Autodesk Fusion 360 part; units mm, degrees
note: some values were not read from the file. Set by a fixed rule: which sketch regions a step uses.
(part 3 of 3)
  arc A1078 (120.8139, 18.409) -> (120.8089, 18.409) centre (120.8114, 18.409) ccw
  arc A1079 (117.7319, 17.663) -> (117.7269, 17.663) centre (117.7294, 17.663) ccw
  arc A1080 (118.5519, 18.189) -> (118.5469, 18.189) centre (118.5494, 18.189) ccw
  arc A1081 (117.9059, 17.837) -> (117.9009, 17.837) centre (117.9034, 17.837) ccw
  arc A1082 (118.7879, 18.242) -> (118.7929, 18.242) centre (118.7904, 18.242) ccw
  arc A1083 (120.8089, 18.409) -> (120.8139, 18.409) centre (120.8114, 18.409) ccw
  arc A1084 (118.5469, 18.189) -> (118.5519, 18.189) centre (118.5494, 18.189) ccw
  line L282 (118.7904, 18.242) -> (119.0274, 18.259)
  line L283 (119.0274, 18.259) -> (119.0364, 18.255)
  arc A1085 (117.4659, 17.248) -> (117.4609, 17.248) centre (117.4634, 17.248) ccw
  line L284 (117.9034, 17.837) -> (118.1014, 17.985)
  arc A1086 (118.3159, 18.103) -> (118.3209, 18.103) centre (118.3184, 18.103) ccw
  line L285 (118.5494, 18.189) -> (118.7904, 18.242)
  line L286 (117.3244, 16.284) -> (117.3774, 16.043)
  arc A1087 (119.0339, 18.255) -> (119.0389, 18.255) centre (119.0364, 18.255) ccw
  arc A1088 (120.0339, 18.255) -> (120.0389, 18.255) centre (120.0364, 18.255) ccw
  arc A1089 (119.0389, 18.255) -> (119.0339, 18.255) centre (119.0364, 18.255) ccw
  arc A1090 (119.0249, 18.259) -> (119.0299, 18.259) centre (119.0274, 18.259) ccw
  arc A1091 (118.3209, 18.103) -> (118.3159, 18.103) centre (118.3184, 18.103) ccw
  arc A1092 (118.3209, 18.103) -> (118.3159, 18.103) centre (118.3184, 18.103) ccw
  arc A1093 (118.3159, 18.103) -> (118.3209, 18.103) centre (118.3184, 18.103) ccw
  arc A1094 (120.2979, 18.272) -> (120.3029, 18.272) centre (120.3004, 18.272) ccw
  arc A1095 (117.7319, 17.663) -> (117.7269, 17.663) centre (117.7294, 17.663) ccw
  arc A1096 (117.9009, 17.837) -> (117.9059, 17.837) centre (117.9034, 17.837) ccw
  arc A1097 (118.0989, 17.985) -> (118.1039, 17.985) centre (118.1014, 17.985) ccw
  arc A1098 (120.0389, 18.255) -> (120.0339, 18.255) centre (120.0364, 18.255) ccw
  arc A1099 (120.5629, 18.324) -> (120.5579, 18.324) centre (120.5604, 18.324) ccw
  arc A1100 (119.0249, 18.259) -> (119.0299, 18.259) centre (119.0274, 18.259) ccw
  line L287 (120.8114, 18.409) -> (121.0484, 18.526)
  arc A1101 (118.0989, 17.985) -> (118.1039, 17.985) centre (118.1014, 17.985) ccw
  arc A1102 (120.2979, 18.272) -> (120.3029, 18.272) centre (120.3004, 18.272) ccw
  arc A1103 (117.5839, 17.465) -> (117.5789, 17.465) centre (117.5814, 17.465) ccw
  line L288 (120.5604, 18.324) -> (120.8114, 18.409)
  line L289 (117.5814, 17.465) -> (117.7294, 17.663)
  arc A1104 (120.3029, 18.272) -> (120.2979, 18.272) centre (120.3004, 18.272) ccw
  arc A1105 (119.0299, 18.259) -> (119.0249, 18.259) centre (119.0274, 18.259) ccw
  arc A1106 (118.5469, 18.189) -> (118.5519, 18.189) centre (118.5494, 18.189) ccw
  arc A1107 (120.8089, 18.409) -> (120.8139, 18.409) centre (120.8114, 18.409) ccw
  line L290 (117.7294, 17.663) -> (117.9034, 17.837)
  arc A1108 (117.7269, 17.663) -> (117.7319, 17.663) centre (117.7294, 17.663) ccw
  arc A1109 (122.0589, 20.28) -> (122.0639, 20.28) centre (122.0614, 20.28) ccw
  arc A1110 (121.9899, 19.7559) -> (121.9949, 19.7559) centre (121.9924, 19.7559) ccw
  arc A1111 (117.9009, 17.837) -> (117.9059, 17.837) centre (117.9034, 17.837) ccw
  arc A1112 (122.0469, 35.2943) -> (122.0419, 35.2943) centre (122.0444, 35.2943) ccw
  arc A1113 (121.9899, 35.5541) -> (121.9949, 35.5541) centre (121.9924, 35.5541) ccw
  arc A1114 (121.4709, 18.8481) -> (121.4659, 18.8481) centre (121.4684, 18.8481) ccw
  arc A1115 (118.7879, 18.242) -> (118.7929, 18.242) centre (118.7904, 18.242) ccw
  arc A1116 (121.6459, 19.0473) -> (121.6409, 19.0473) centre (121.6434, 19.0473) ccw
  arc A1117 (122.0639, 35.03) -> (122.0589, 35.03) centre (122.0614, 35.03) ccw
  arc A1118 (121.9949, 35.5541) -> (121.9899, 35.5541) centre (121.9924, 35.5541) ccw
  arc A1119 (121.9899, 35.5541) -> (121.9949, 35.5541) centre (121.9924, 35.5541) ccw
  arc A1120 (121.7879, 19.2675) -> (121.7929, 19.2675) centre (121.7904, 19.2675) ccw
  arc A1121 (121.0509, 18.526) -> (121.0459, 18.526) centre (121.0484, 18.526) ccw
  line L291 (121.6434, 19.0473) -> (121.7904, 19.2675)
  arc A1122 (122.0419, 20.0157) -> (122.0469, 20.0157) centre (122.0444, 20.0157) ccw
  arc A1123 (122.0589, 35.03) -> (122.0639, 35.03) centre (122.0614, 35.03) ccw
  arc A1124 (121.7879, 36.0425) -> (121.7929, 36.0425) centre (121.7904, 36.0425) ccw
  arc A1125 (118.1039, 17.985) -> (118.0989, 17.985) centre (118.1014, 17.985) ccw
  arc A1126 (121.6409, 19.0473) -> (121.6459, 19.0473) centre (121.6434, 19.0473) ccw
  arc A1127 (121.2669, 18.6735) -> (121.2719, 18.6735) centre (121.2694, 18.6735) ccw
  line L292 (120.0364, 18.255) -> (120.3004, 18.272)
  arc A1128 (121.0509, 18.526) -> (121.0459, 18.526) centre (121.0484, 18.526) ccw
  arc A1129 (121.6459, 19.0473) -> (121.6409, 19.0473) centre (121.6434, 19.0473) ccw
  arc A1130 (121.9099, 19.5051) -> (121.9049, 19.5051) centre (121.9074, 19.5051) ccw
  arc A1131 (121.9949, 19.7559) -> (121.9899, 19.7559) centre (121.9924, 19.7559) ccw
  line L293 (122.0614, 20.28) -> (122.0614, 35.03)
  arc A1132 (122.0419, 35.2943) -> (122.0469, 35.2943) centre (122.0444, 35.2943) ccw
  arc A1133 (121.9949, 35.5541) -> (121.9899, 35.5541) centre (121.9924, 35.5541) ccw
  line L294 (122.0444, 35.2943) -> (122.0614, 35.03)
  arc A1134 (121.7929, 19.2675) -> (121.7879, 19.2675) centre (121.7904, 19.2675) ccw
  arc A1135 (121.9949, 19.7559) -> (121.9899, 19.7559) centre (121.9924, 19.7559) ccw
  line L295 (121.7904, 36.0425) -> (121.9074, 35.8049)
  line L296 (121.9924, 19.7559) -> (122.0444, 20.0157)
  line L297 (121.9074, 35.8049) -> (121.9924, 35.5541)
  arc A1136 (122.0469, 20.0157) -> (122.0419, 20.0157) centre (122.0444, 20.0157) ccw
  arc A1137 (121.0459, 18.526) -> (121.0509, 18.526) centre (121.0484, 18.526) ccw
  arc A1138 (122.0639, 35.03) -> (122.0589, 35.03) centre (122.0614, 35.03) ccw
  arc A1139 (121.7879, 19.2675) -> (121.7929, 19.2675) centre (121.7904, 19.2675) ccw
  arc A1140 (121.9049, 35.8049) -> (121.9099, 35.8049) centre (121.9074, 35.8049) ccw
  arc A1141 (121.9099, 35.8049) -> (121.9049, 35.8049) centre (121.9074, 35.8049) ccw
  line L298 (121.7904, 19.2675) -> (121.9074, 19.5051)
  arc A1142 (117.5789, 17.465) -> (117.5839, 17.465) centre (117.5814, 17.465) ccw
  line L299 (118.3184, 18.103) -> (118.5494, 18.189)
  arc A1143 (121.9049, 19.5051) -> (121.9099, 19.5051) centre (121.9074, 19.5051) ccw
  arc A1144 (121.9049, 19.5051) -> (121.9099, 19.5051) centre (121.9074, 19.5051) ccw
  arc A1145 (122.0419, 35.2943) -> (122.0469, 35.2943) centre (122.0444, 35.2943) ccw
  line L300 (121.9924, 35.5541) -> (122.0444, 35.2943)
  arc A1146 (121.6409, 19.0473) -> (121.6459, 19.0473) centre (121.6434, 19.0473) ccw
  line L301 (121.4684, 18.8481) -> (121.6434, 19.0473)
  arc A1147 (119.0339, 18.255) -> (119.0389, 18.255) centre (119.0364, 18.255) ccw
  arc A1148 (122.0589, 35.03) -> (122.0639, 35.03) centre (122.0614, 35.03) ccw
  arc A1149 (122.0469, 35.2943) -> (122.0419, 35.2943) centre (122.0444, 35.2943) ccw
  arc A1150 (121.4659, 18.8481) -> (121.4709, 18.8481) centre (121.4684, 18.8481) ccw
  line L302 (121.2694, 18.6735) -> (121.4684, 18.8481)
  arc A1151 (118.7929, 18.242) -> (118.7879, 18.242) centre (118.7904, 18.242) ccw
  arc A1152 (121.0459, 18.526) -> (121.0509, 18.526) centre (121.0484, 18.526) ccw
  arc A1153 (121.6409, 36.2627) -> (121.6459, 36.2627) centre (121.6434, 36.2627) ccw
  arc A1154 (120.8139, 36.9009) -> (120.8089, 36.9009) centre (120.8114, 36.9009) ccw
  arc A1155 (121.4709, 18.8481) -> (121.4659, 18.8481) centre (121.4684, 18.8481) ccw
  arc A1156 (121.4709, 36.4619) -> (121.4659, 36.4619) centre (121.4684, 36.4619) ccw
  arc A1157 (120.8089, 36.9009) -> (120.8139, 36.9009) centre (120.8114, 36.9009) ccw
  line L303 (57.5614, 30.53) -> (57.5614, 32.53)
  line L304 (122.0444, 20.0157) -> (122.0614, 20.28)
  arc A1158 (121.0509, 36.7837) -> (121.0459, 36.7837) centre (121.0484, 36.7837) ccw
  line L305 (121.0484, 36.7837) -> (121.2694, 36.6365)
  arc A1159 (122.0469, 20.0157) -> (122.0419, 20.0157) centre (122.0444, 20.0157) ccw
  arc A1160 (121.2719, 18.6735) -> (121.2669, 18.6735) centre (121.2694, 18.6735) ccw
  arc A1161 (120.5629, 36.986) -> (120.5579, 36.986) centre (120.5604, 36.986) ccw
  arc A1162 (121.6409, 36.2627) -> (121.6459, 36.2627) centre (121.6434, 36.2627) ccw
  line L306 (57.5439, 32.7183) -> (57.5614, 32.53)
  line L307 (121.0484, 18.526) -> (121.2694, 18.6735)
  arc A1163 (121.9049, 35.8049) -> (121.9099, 35.8049) centre (121.9074, 35.8049) ccw
  arc A1164 (121.4709, 36.4619) -> (121.4659, 36.4619) centre (121.4684, 36.4619) ccw
  arc A1165 (57.5589, 32.53) -> (57.5639, 32.53) centre (57.5614, 32.53) ccw
  arc A1166 (121.4659, 36.4619) -> (121.4709, 36.4619) centre (121.4684, 36.4619) ccw
  arc A1167 (121.9099, 35.8049) -> (121.9049, 35.8049) centre (121.9074, 35.8049) ccw
  arc A1168 (120.8089, 36.9009) -> (120.8139, 36.9009) centre (120.8114, 36.9009) ccw
  arc A1169 (121.7879, 36.0425) -> (121.7929, 36.0425) centre (121.7904, 36.0425) ccw
  arc A1170 (121.2669, 36.6365) -> (121.2719, 36.6365) centre (121.2694, 36.6365) ccw
  line L308 (121.2694, 36.6365) -> (121.4684, 36.4619)
  arc A1171 (57.5639, 32.53) -> (57.5589, 32.53) centre (57.5614, 32.53) ccw
  arc A1172 (121.7929, 36.0425) -> (121.7879, 36.0425) centre (121.7904, 36.0425) ccw
  arc A1173 (121.2669, 18.6735) -> (121.2719, 18.6735) centre (121.2694, 18.6735) ccw
  arc A1174 (121.2719, 18.6735) -> (121.2669, 18.6735) centre (121.2694, 18.6735) ccw
  arc A1175 (122.0589, 20.28) -> (122.0639, 20.28) centre (122.0614, 20.28) ccw
  arc A1176 (57.5589, 30.53) -> (57.5639, 30.53) centre (57.5614, 30.53) ccw
  arc A1177 (57.5589, 32.53) -> (57.5639, 32.53) centre (57.5614, 32.53) ccw
  arc A1178 (57.5464, 32.7183) -> (57.5414, 32.7183) centre (57.5439, 32.7183) ccw
  arc A1179 (121.7929, 19.2675) -> (121.7879, 19.2675) centre (121.7904, 19.2675) ccw
  arc A1180 (122.0419, 20.0157) -> (122.0469, 20.0157) centre (122.0444, 20.0157) ccw
  arc A1181 (121.9899, 19.7559) -> (121.9949, 19.7559) centre (121.9924, 19.7559) ccw
  arc A1182 (120.8139, 36.9009) -> (120.8089, 36.9009) centre (120.8114, 36.9009) ccw
  line L309 (120.5604, 36.986) -> (120.8114, 36.9009)
  arc A1183 (121.2669, 36.6365) -> (121.2719, 36.6365) centre (121.2694, 36.6365) ccw
  arc A1184 (121.6459, 36.2627) -> (121.6409, 36.2627) centre (121.6434, 36.2627) ccw
  arc A1185 (122.0639, 20.28) -> (122.0589, 20.28) centre (122.0614, 20.28) ccw
  arc A1186 (57.5639, 30.53) -> (57.5589, 30.53) centre (57.5614, 30.53) ccw
  arc A1187 (121.0459, 36.7837) -> (121.0509, 36.7837) centre (121.0484, 36.7837) ccw
  arc A1188 (121.4659, 18.8481) -> (121.4709, 18.8481) centre (121.4684, 18.8481) ccw
  arc A1189 (121.7929, 36.0425) -> (121.7879, 36.0425) centre (121.7904, 36.0425) ccw
  arc A1190 (121.6459, 36.2627) -> (121.6409, 36.2627) centre (121.6434, 36.2627) ccw
  line L310 (120.8114, 36.9009) -> (121.0484, 36.7837)
  line L311 (121.4684, 36.4619) -> (121.6434, 36.2627)
  arc A1191 (121.4659, 36.4619) -> (121.4709, 36.4619) centre (121.4684, 36.4619) ccw
  line L312 (121.9074, 19.5051) -> (121.9924, 19.7559)
  arc A1192 (121.9099, 19.5051) -> (121.9049, 19.5051) centre (121.9074, 19.5051) ccw
  line L313 (121.6434, 36.2627) -> (121.7904, 36.0425)
  arc A1193 (122.0639, 20.28) -> (122.0589, 20.28) centre (122.0614, 20.28) ccw
  arc A1194 (121.0509, 36.7837) -> (121.0459, 36.7837) centre (121.0484, 36.7837) ccw
  arc A1195 (121.2719, 36.6365) -> (121.2669, 36.6365) centre (121.2694, 36.6365) ccw
  arc A1196 (120.5579, 36.986) -> (120.5629, 36.986) centre (120.5604, 36.986) ccw
  arc A1197 (121.0459, 36.7837) -> (121.0509, 36.7837) centre (121.0484, 36.7837) ccw
  arc A1198 (121.2719, 36.6365) -> (121.2669, 36.6365) centre (121.2694, 36.6365) ccw
  arc A1199 (57.5639, 32.53) -> (57.5589, 32.53) centre (57.5614, 32.53) ccw
  arc A1200 (56.9908, 33.4475) -> (56.9958, 33.4475) centre (56.9933, 33.4475) ccw
  line L314 (64.9184, 33.348) -> (65.0794, 33.4475)
  arc A1201 (65.6339, 33.5506) -> (65.6289, 33.5506) centre (65.6314, 33.5506) ccw
  arc A1202 (65.0769, 33.4475) -> (65.0819, 33.4475) centre (65.0794, 33.4475) ccw
  arc A1203 (65.0819, 33.4475) -> (65.0769, 33.4475) centre (65.0794, 33.4475) ccw
  arc A1204 (64.9159, 33.348) -> (64.9209, 33.348) centre (64.9184, 33.348) ccw
  arc A1205 (64.9209, 33.348) -> (64.9159, 33.348) centre (64.9184, 33.348) ccw
  arc A1206 (65.2529, 33.5159) -> (65.2579, 33.5159) centre (65.2554, 33.5159) ccw
  line L315 (65.4414, 33.5506) -> (65.6314, 33.5506)
  arc A1207 (65.4439, 33.5506) -> (65.4389, 33.5506) centre (65.4414, 33.5506) ccw
  arc A1208 (57.2964, 33.2205) -> (57.2914, 33.2205) centre (57.2939, 33.2205) ccw
  arc A1209 (56.9958, 33.4475) -> (56.9908, 33.4475) centre (56.9933, 33.4475) ccw
  arc A1210 (65.2579, 33.5159) -> (65.2529, 33.5159) centre (65.2554, 33.5159) ccw
  line L316 (57.4922, 32.9003) -> (57.5439, 32.7183)
  arc A1211 (57.2914, 33.2205) -> (57.2964, 33.2205) centre (57.2939, 33.2205) ccw
  arc A1212 (57.2914, 33.2205) -> (57.2964, 33.2205) centre (57.2939, 33.2205) ccw
  arc A1213 (65.0769, 33.4475) -> (65.0819, 33.4475) centre (65.0794, 33.4475) ccw
  arc A1214 (57.5414, 32.7183) -> (57.5464, 32.7183) centre (57.5439, 32.7183) ccw
  arc A1215 (57.4947, 32.9003) -> (57.4897, 32.9003) centre (57.4922, 32.9003) ccw
  arc A1216 (56.9958, 33.4475) -> (56.9908, 33.4475) centre (56.9933, 33.4475) ccw
  line L317 (57.2939, 33.2205) -> (57.4079, 33.0696)
  arc A1217 (57.1566, 33.348) -> (57.1516, 33.348) centre (57.1541, 33.348) ccw
  arc A1218 (65.0819, 33.4475) -> (65.0769, 33.4475) centre (65.0794, 33.4475) ccw
  line L318 (64.7794, 33.2205) -> (64.9184, 33.348)
  arc A1219 (64.7769, 33.2205) -> (64.7819, 33.2205) centre (64.7794, 33.2205) ccw
  arc A1220 (57.5464, 32.7183) -> (57.5414, 32.7183) centre (57.5439, 32.7183) ccw
  line L319 (56.9933, 33.4475) -> (57.1541, 33.348)
  arc A1221 (65.6289, 33.5506) -> (65.6339, 33.5506) centre (65.6314, 33.5506) ccw
  line L320 (57.1541, 33.348) -> (57.2939, 33.2205)
  line L321 (56.8169, 33.5159) -> (56.9933, 33.4475)
  arc A1222 (65.4389, 33.5506) -> (65.4439, 33.5506) centre (65.4414, 33.5506) ccw
  arc A1223 (65.4439, 33.5506) -> (65.4389, 33.5506) centre (65.4414, 33.5506) ccw
  arc A1224 (57.4054, 33.0696) -> (57.4104, 33.0696) centre (57.4079, 33.0696) ccw
  arc A1225 (65.6339, 33.5506) -> (65.6289, 33.5506) centre (65.6314, 33.5506) ccw
  arc A1226 (65.8149, 33.5159) -> (65.8199, 33.5159) centre (65.8174, 33.5159) ccw
  arc A1227 (65.2529, 33.5159) -> (65.2579, 33.5159) centre (65.2554, 33.5159) ccw
  arc A1228 (57.4054, 33.0696) -> (57.4104, 33.0696) centre (57.4079, 33.0696) ccw
  line L322 (65.2554, 33.5159) -> (65.4414, 33.5506)
  arc A1229 (57.1516, 33.348) -> (57.1566, 33.348) centre (57.1541, 33.348) ccw
  line L323 (65.0794, 33.4475) -> (65.2554, 33.5159)
  arc A1230 (57.4104, 33.0696) -> (57.4054, 33.0696) centre (57.4079, 33.0696) ccw
  arc A1231 (57.1516, 33.348) -> (57.1566, 33.348) centre (57.1541, 33.348) ccw
  arc A1232 (57.4947, 32.9003) -> (57.4897, 32.9003) centre (57.4922, 32.9003) ccw
  arc A1233 (56.9908, 33.4475) -> (56.9958, 33.4475) centre (56.9933, 33.4475) ccw
  arc A1234 (56.8194, 33.5159) -> (56.8144, 33.5159) centre (56.8169, 33.5159) ccw
  arc A1235 (65.8199, 33.5159) -> (65.8149, 33.5159) centre (65.8174, 33.5159) ccw
  arc A1236 (57.5414, 32.7183) -> (57.5464, 32.7183) centre (57.5439, 32.7183) ccw
  arc A1237 (57.4104, 33.0696) -> (57.4054, 33.0696) centre (57.4079, 33.0696) ccw
  arc A1238 (56.8144, 33.5159) -> (56.8194, 33.5159) centre (56.8169, 33.5159) ccw
  line L324 (65.6314, 33.5506) -> (65.8174, 33.5159)
  arc A1239 (57.4897, 32.9003) -> (57.4947, 32.9003) centre (57.4922, 32.9003) ccw
  arc A1240 (65.4389, 33.5506) -> (65.4439, 33.5506) centre (65.4414, 33.5506) ccw
  arc A1241 (65.2579, 33.5159) -> (65.2529, 33.5159) centre (65.2554, 33.5159) ccw
  arc A1242 (65.6289, 33.5506) -> (65.6339, 33.5506) centre (65.6314, 33.5506) ccw
  line L325 (57.4079, 33.0696) -> (57.4922, 32.9003)
  arc A1243 (57.4897, 32.9003) -> (57.4947, 32.9003) centre (57.4922, 32.9003) ccw
  arc A1244 (57.2964, 33.2205) -> (57.2914, 33.2205) centre (57.2939, 33.2205) ccw
  arc A1245 (57.1566, 33.348) -> (57.1516, 33.348) centre (57.1541, 33.348) ccw
  arc A1246 (55.9212, 33.348) -> (55.9162, 33.348) centre (55.9187, 33.348) ccw
  arc A1247 (55.6674, 33.0696) -> (55.6624, 33.0696) centre (55.6649, 33.0696) ccw
  arc A1248 (64.5309, 32.7183) -> (64.5259, 32.7183) centre (64.5284, 32.7183) ccw
  arc A1249 (64.7819, 33.2205) -> (64.7769, 33.2205) centre (64.7794, 33.2205) ccw
  arc A1250 (56.6285, 33.5506) -> (56.6335, 33.5506) centre (56.631, 33.5506) ccw
  arc A1251 (56.077, 33.4475) -> (56.082, 33.4475) centre (56.0795, 33.4475) ccw
  arc A1252 (56.2534, 33.5159) -> (56.2584, 33.5159) centre (56.2559, 33.5159) ccw
  arc A1253 (64.7769, 33.2205) -> (64.7819, 33.2205) centre (64.7794, 33.2205) ccw
  arc A1254 (55.7764, 33.2205) -> (55.7814, 33.2205) centre (55.7789, 33.2205) ccw
  line L326 (55.9187, 33.348) -> (56.0795, 33.4475)
  arc A1255 (56.4443, 33.5506) -> (56.4393, 33.5506) centre (56.4418, 33.5506) ccw
  line L327 (56.2559, 33.5159) -> (56.4418, 33.5506)
  line L328 (64.6654, 33.0696) -> (64.7794, 33.2205)
  arc A1256 (64.9209, 33.348) -> (64.9159, 33.348) centre (64.9184, 33.348) ccw
  arc A1257 (56.8194, 33.5159) -> (56.8144, 33.5159) centre (56.8169, 33.5159) ccw
  arc A1258 (56.4443, 33.5506) -> (56.4393, 33.5506) centre (56.4418, 33.5506) ccw
  arc A1259 (56.077, 33.4475) -> (56.082, 33.4475) centre (56.0795, 33.4475) ccw
  arc A1260 (64.7819, 33.2205) -> (64.7769, 33.2205) centre (64.7794, 33.2205) ccw
  line L329 (56.4418, 33.5506) -> (56.631, 33.5506)
  arc A1261 (56.2584, 33.5159) -> (56.2534, 33.5159) centre (56.2559, 33.5159) ccw
  arc A1262 (55.7814, 33.2205) -> (55.7764, 33.2205) centre (55.7789, 33.2205) ccw
  arc A1263 (55.9162, 33.348) -> (55.9212, 33.348) centre (55.9187, 33.348) ccw
  arc A1264 (56.082, 33.4475) -> (56.077, 33.4475) centre (56.0795, 33.4475) ccw
  arc A1265 (56.4393, 33.5506) -> (56.4443, 33.5506) centre (56.4418, 33.5506) ccw
  arc A1266 (56.2534, 33.5159) -> (56.2584, 33.5159) centre (56.2559, 33.5159) ccw
  arc A1267 (55.6674, 33.0696) -> (55.6624, 33.0696) centre (55.6649, 33.0696) ccw
  arc A1268 (64.5259, 32.7183) -> (64.5309, 32.7183) centre (64.5284, 32.7183) ccw
  arc A1269 (55.5264, 32.7183) -> (55.5314, 32.7183) centre (55.5289, 32.7183) ccw
  arc A1270 (55.5781, 32.9003) -> (55.5831, 32.9003) centre (55.5806, 32.9003) ccw
  arc A1271 (56.4393, 33.5506) -> (56.4443, 33.5506) centre (56.4418, 33.5506) ccw
  arc A1272 (55.6624, 33.0696) -> (55.6674, 33.0696) centre (55.6649, 33.0696) ccw
  arc A1273 (64.5779, 32.9003) -> (64.5829, 32.9003) centre (64.5804, 32.9003) ccw
  line L330 (55.7789, 33.2205) -> (55.9187, 33.348)
  line L331 (56.0795, 33.4475) -> (56.2559, 33.5159)
  arc A1274 (57.5639, 30.53) -> (57.5589, 30.53) centre (57.5614, 30.53) ccw
  arc A1275 (57.5589, 30.53) -> (57.5639, 30.53) centre (57.5614, 30.53) ccw
  arc A1276 (55.9162, 33.348) -> (55.9212, 33.348) centre (55.9187, 33.348) ccw
  arc A1277 (56.6335, 33.5506) -> (56.6285, 33.5506) centre (56.631, 33.5506) ccw
  arc A1278 (56.2584, 33.5159) -> (56.2534, 33.5159) centre (56.2559, 33.5159) ccw
  arc A1279 (56.082, 33.4475) -> (56.077, 33.4475) centre (56.0795, 33.4475) ccw
  arc A1280 (55.7764, 33.2205) -> (55.7814, 33.2205) centre (55.7789, 33.2205) ccw
  arc A1281 (64.6679, 33.0696) -> (64.6629, 33.0696) centre (64.6654, 33.0696) ccw
  arc A1282 (64.9159, 33.348) -> (64.9209, 33.348) centre (64.9184, 33.348) ccw
  arc A1283 (64.5829, 32.9003) -> (64.5779, 32.9003) centre (64.5804, 32.9003) ccw
  line L332 (64.5284, 32.7183) -> (64.5804, 32.9003)
  arc A1284 (64.6629, 33.0696) -> (64.6679, 33.0696) centre (64.6654, 33.0696) ccw
  arc A1285 (55.9212, 33.348) -> (55.9162, 33.348) centre (55.9187, 33.348) ccw
  arc A1286 (55.7814, 33.2205) -> (55.7764, 33.2205) centre (55.7789, 33.2205) ccw
  arc A1287 (55.5781, 32.9003) -> (55.5831, 32.9003) centre (55.5806, 32.9003) ccw
  arc A1288 (55.5831, 32.9003) -> (55.5781, 32.9003) centre (55.5806, 32.9003) ccw
  arc A1289 (64.6629, 33.0696) -> (64.6679, 33.0696) centre (64.6654, 33.0696) ccw
  arc A1290 (64.6679, 33.0696) -> (64.6629, 33.0696) centre (64.6654, 33.0696) ccw
  arc A1291 (64.5779, 32.9003) -> (64.5829, 32.9003) centre (64.5804, 32.9003) ccw
  arc A1292 (57.5464, 30.3417) -> (57.5414, 30.3417) centre (57.5439, 30.3417) ccw
  line L333 (55.6649, 33.0696) -> (55.7789, 33.2205)
  line L334 (64.5804, 32.9003) -> (64.6654, 33.0696)
  arc A1293 (57.5414, 30.3417) -> (57.5464, 30.3417) centre (57.5439, 30.3417) ccw
  line L335 (107.7904, 1.018) -> (107.9074, 1.255)
  arc A1294 (108.0769, 3.288) -> (108.0719, 3.288) centre (108.0744, 3.288) ccw
  arc A1295 (108.1219, 3.542) -> (108.1269, 3.542) centre (108.1244, 3.542) ccw
  circle A1296 centre (12.7254, 3.937) radius 0.45 construction
  line L336 (11.8504, 5.602) -> (11.8504, 7.352) construction
  line L337 (13.6004, 5.602) -> (11.8504, 5.602) construction
  line L338 (27.5938, 3.7375) -> (27.5938, 5.5875) construction
  line L339 (29.4438, 3.7375) -> (27.5938, 3.7375) construction
  circle A1297 centre (28.5188, 4.6625) radius 0.5 construction
  circle A1298 centre (26.0188, 4.6625) radius 0.925 construction
  circle A1299 centre (12.7254, 6.477) radius 0.45 construction
  circle A1300 centre (72.7364, 31.0857) radius 1.225 construction
  circle A1301 centre (77.7364, 31.0857) radius 1.225 construction
  circle A1302 centre (10.1854, 6.477) radius 0.875 construction
  circle A1303 centre (10.1854, 3.937) radius 0.875 construction
  circle A1304 centre (43.897, 31.0857) radius 1.225 construction
  circle A1305 centre (48.897, 31.0857) radius 0.7 construction
  circle A1306 centre (10.1854, 3.937) radius 0.45 construction
  circle A1307 centre (48.897, 31.0857) radius 1.225 construction
  circle A1308 centre (10.1854, 6.477) radius 0.45 construction
  circle A1309 centre (77.7364, 31.0857) radius 0.7 construction
  line L340 (11.8504, 7.352) -> (13.6004, 7.352) construction
  circle A1310 centre (35.3679, 34.0015) radius 0.875 construction
  circle A1311 centre (8.4979, 19.224) radius 0.925 construction
  line L341 (13.6004, 7.352) -> (13.6004, 5.602) construction
  line L342 (7.5729, 15.149) -> (9.4229, 15.149) construction
  line L343 (37.0329, 34.8765) -> (38.7829, 34.8765) construction
  line L344 (9.4229, 15.149) -> (9.4229, 13.299) construction
  line L345 (9.4229, 13.299) -> (7.5729, 13.299) construction
  circle A1312 centre (35.3679, 31.4615) radius 0.45 construction
  line L346 (28.3943, 33.0249) -> (26.6443, 33.0249) construction
  circle A1313 centre (37.9079, 34.0015) radius 0.45 construction
  line L347 (7.5729, 13.299) -> (7.5729, 15.149) construction
  circle A1314 centre (8.4979, 16.724) radius 0.925 construction
  circle A1315 centre (43.897, 31.0857) radius 0.7 construction
  circle A1316 centre (23.5188, 4.6625) radius 0.5 construction
  circle A1317 centre (12.7254, 3.937) radius 0.875 construction
  circle A1318 centre (8.4979, 14.224) radius 0.5 construction
  circle A1319 centre (72.7364, 31.0857) radius 0.7 construction
  circle A1320 centre (23.5188, 4.6625) radius 0.925 construction
  line L348 (38.7829, 34.8765) -> (38.7829, 33.1265) construction
  circle A1321 centre (35.3679, 34.0015) radius 0.45 construction
  line L349 (29.4438, 5.5875) -> (29.4438, 3.7375) construction
  circle A1322 centre (26.0188, 4.6625) radius 0.5 construction
  line L350 (37.0329, 33.1265) -> (37.0329, 34.8765) construction
  circle A1323 centre (27.5193, 31.3599) radius 0.45 construction
  line L351 (38.7829, 33.1265) -> (37.0329, 33.1265) construction
  circle A1324 centre (8.4979, 19.224) radius 0.5 construction
  circle A1325 centre (35.3679, 31.4615) radius 0.875 construction
  circle A1326 centre (24.9793, 33.8999) radius 0.875 construction
  circle A1327 centre (8.4979, 21.724) radius 0.925 construction
  line L352 (27.5938, 5.5875) -> (29.4438, 5.5875) construction
  arc A1328 (83.6167, 10.5889) -> (84.2667, 10.5889) centre (83.9417, 10.5889) ccw construction
  arc A1329 (83.3167, 10.6139) -> (84.5667, 10.6139) centre (83.9417, 10.6139) ccw construction
  arc A1330 (79.9067, 6.3739) -> (78.6567, 6.3739) centre (79.2817, 6.3739) ccw construction
  circle A1331 centre (8.4979, 16.724) radius 0.5 construction
  line L353 (26.6443, 33.0249) -> (26.6443, 34.7749) construction
  circle A1332 centre (112.7141, 21.9272) radius 0.925 construction
  circle A1333 centre (24.9793, 31.3599) radius 0.875 construction
  line L354 (113.6391, 13.5022) -> (111.7891, 13.5022) construction
  circle A1334 centre (81.6116, 12.4939) radius 0.35 construction
  line L355 (78.6567, 6.3739) -> (78.6567, 5.8739) construction
  line L356 (43.1948, 5.6637) -> (45.0448, 5.6637) construction
  circle A1335 centre (37.9079, 31.4615) radius 0.45 construction
  circle A1336 centre (36.6198, 4.7387) radius 0.925 construction
  circle A1337 centre (27.5193, 31.3599) radius 0.875 construction
  circle A1338 centre (39.1198, 4.7387) radius 0.925 construction
  line L357 (26.6443, 34.7749) -> (28.3943, 34.7749) construction
  line L358 (28.3943, 34.7749) -> (28.3943, 33.0249) construction
  line L359 (45.0448, 3.8137) -> (43.1948, 3.8137) construction
  circle A1339 centre (36.6198, 4.7387) radius 0.5 construction
  line L360 (111.7891, 15.3522) -> (113.6391, 15.3522) construction
  circle A1340 centre (27.5193, 33.8999) radius 0.45 construction
  line L361 (111.7891, 13.5022) -> (111.7891, 15.3522) construction
  circle A1341 centre (24.9793, 33.8999) radius 0.45 construction
  arc A1342 (78.6567, 5.8739) -> (79.9067, 5.8739) centre (79.2817, 5.8739) ccw construction
  circle A1343 centre (112.7141, 16.9272) radius 0.5 construction
  arc A1344 (78.9567, 5.8489) -> (79.6067, 5.8489) centre (79.2817, 5.8489) ccw construction
  circle A1345 centre (112.7141, 14.4272) radius 0.5 construction
  circle A1346 centre (81.6116, 4.4939) radius 0.35 construction
  circle A1347 centre (112.7141, 21.9272) radius 0.5 construction
  circle A1348 centre (24.9793, 31.3599) radius 0.45 construction
  line L362 (113.6391, 15.3522) -> (113.6391, 13.5022) construction
  line L363 (79.9067, 5.8739) -> (79.9067, 6.3739) construction
  circle A1349 centre (112.7141, 16.9272) radius 0.925 construction
  circle A1350 centre (112.7141, 19.4272) radius 0.925 construction
  circle A1351 centre (112.7141, 19.4272) radius 0.5 construction
  circle A1352 centre (81.6116, 4.4939) radius 0.475 construction
  circle A1353 centre (39.1198, 4.7387) radius 0.5 construction
  circle A1354 centre (44.1198, 4.7387) radius 0.5 construction
  circle A1355 centre (8.4979, 21.724) radius 0.5 construction
  line L364 (43.1948, 3.8137) -> (43.1948, 5.6637) construction
  line L365 (45.0448, 5.6637) -> (45.0448, 3.8137) construction
  line L366 (79.9067, 10.6139) -> (79.9067, 11.1139) construction
  circle A1356 centre (37.9079, 31.4615) radius 0.875 construction
  circle A1357 centre (41.6198, 4.7387) radius 0.5 construction
  circle A1358 centre (41.6198, 4.7387) radius 0.925 construction
  circle A1359 centre (81.6116, 12.4939) radius 0.475 construction
  arc A1360 (84.2667, 6.3989) -> (83.6167, 6.3989) centre (83.9417, 6.3989) ccw construction
  arc A1361 (84.2667, 11.1389) -> (83.6167, 11.1389) centre (83.9417, 11.1389) ccw construction
  line L367 (84.2667, 10.5889) -> (84.2667, 11.1389) construction
  arc A1362 (78.9567, 10.5889) -> (79.6067, 10.5889) centre (79.2817, 10.5889) ccw construction
  line L368 (78.6567, 11.1139) -> (78.6567, 10.6139) construction
  line L369 (84.5667, 5.8739) -> (84.5667, 6.3739) construction
  line L370 (79.6067, 5.8489) -> (79.6067, 6.3989) construction
  line L371 (83.3167, 6.3739) -> (83.3167, 5.8739) construction
  arc A1363 (84.5667, 11.1139) -> (83.3167, 11.1139) centre (83.9417, 11.1139) ccw construction
  arc A1364 (78.6567, 10.6139) -> (79.9067, 10.6139) centre (79.2817, 10.6139) ccw construction
  arc A1365 (79.6067, 6.3989) -> (78.9567, 6.3989) centre (79.2817, 6.3989) ccw construction
  arc A1366 (79.9067, 11.1139) -> (78.6567, 11.1139) centre (79.2817, 11.1139) ccw construction
  line L372 (78.9567, 11.1389) -> (78.9567, 10.5889) construction
  line L373 (83.3167, 11.1139) -> (83.3167, 10.6139) construction
  arc A1367 (84.5667, 6.3739) -> (83.3167, 6.3739) centre (83.9417, 6.3739) ccw construction
  line L374 (78.9567, 6.3989) -> (78.9567, 5.8489) construction
  line L375 (79.6067, 10.5889) -> (79.6067, 11.1389) construction
  line L376 (84.2667, 5.8489) -> (84.2667, 6.3989) construction
  line L377 (83.6167, 6.3989) -> (83.6167, 5.8489) construction
  line L378 (83.6167, 11.1389) -> (83.6167, 10.5889) construction
  arc A1368 (79.6067, 11.1389) -> (78.9567, 11.1389) centre (79.2817, 11.1389) ccw construction
  arc A1369 (83.6167, 5.8489) -> (84.2667, 5.8489) centre (83.9417, 5.8489) ccw construction
  arc A1370 (83.3167, 5.8739) -> (84.5667, 5.8739) centre (83.9417, 5.8739) ccw construction
  line L379 (84.5667, 10.6139) -> (84.5667, 11.1139) construction
extrude "Extrude1" add sketch "Sketch1" against normal blind 3.2 contours A0 A27 A60 A624 | A53 A76 A89 A111 | A29 A38 A40 A61 | A90 A116 A135 A136 | A69 A86 A107 A143 | A94 A106 A134 A155 | A95 A108 A124 A128 | A91 A96 A114 A138 | A87 A118 A139 A156 | A113 A123 A145 A153 | A726 A735 A783 A790 A792 A795 A807 A809 | A772 A782 A800 A813 | A770 A822 A827 A835 | A786 A833 A842 A853 | A787 A829 A846 A864 | A811 A825 A852 A854 | A880 A881 A895 A896 | A848 A869 A879 A904 | A850 A878 A890 A911 | A875 A883 A888 A908 | A840 A899 A903 A905 | A844 A884 A900 A902 | A867 A876 A898 A907 | A516 A541 A550 A564 | A522 A525 A529 A530 A538 A546 A548 A549 | A514 A527 A537 A545 | A521 A534 A535 A547 | A526 A553 A554 A561 | A556 A557 A562 A620 | A582 A607 A608 A614 | A595 A605 A611 A613 | A563 A593 A610 A616 | A566 A571 A596 A597 | L12 L13 L14 L15 L16 L17 L18 L19 L20 L22 L23 L24 L25 L26 L27 L28 L29 L30 L31 L32 L33 L34 L35 L36 L37 L38 L39 L40 L41 L42 L43 L44 L45 L46 L47 L48 L49 L50 L51 L79 L80 L81 L82 L83 L85 L86 L87 L88 L89 L90 L91 L92 L93 L94 L95 L96 L97 L98 L99 L100 L101 L102 L103 L104 L105 L106 L107 L108 L109 L110 L111 L112 L113 L114 L116 L117 L118 L119 L120 L121 L122 L123 L124 L125 L126 L127 L128 L129 L130 L131 L132 L133 L134 L135 L136 L137 L138 L139 L140 L141 L142 L143 L145 L146 L147 L148 L149 L150 L151 L152 L153 L154 L155 L156 L157 L158 L159 L160 L161 L162 L163 L164 L165 L166 L167 L168 L169 L188 L193 L195 L196 L198 L199 L200 L201 L202 L203 L204 L205 L206 L207 L208 L209 L210 L211 L212 L213 L214 L215 L217 L219 L220 L221 L222 L223 L224 L225 L226 L227 L228 L229 L230 L231 L232 L233 L234 L235 L236 L237 L238 L239 L240 L241 L242 L243 L244 L245 L246 L247 L248 L249 L250 L251 L252 L253 L254 L255 L256 L258 L259 L260 L261 L262 L263 L264 L265 L266 L267 L268 L269 L270 L271 L272 L273 L274 L275 L276 L277 L278 L279 L280 L281 L282 L284 L285 L286 L287 L288 L289 L290 L291 L292 L293 L294 L295 L296 L297 L298 L299 L300 L301 L302 L304 L305 L307 L308 L309 L310 L311 L312 L313 L335 | A572 A577 A602 A603 | A573 A585 A617 A621 | A575 A579 A587 A592 | A469 A474 A500 A505 | A479 A499 A507 A544 | A477 A486 A491 A513 | A464 A466 A509 A519 | A489 A490 A501 A543 | A482 A487 A493 A536 | A414 A476 A480 A481 | A441 A458 A488 A523 | A450 A456 A494 A495 | A411 A427 A449 A460 | A430 A454 A459 A504 | A416 A423 A433 A447 | A431 A435 A453 A508 | A319 A324 A330 A337 | A314 A329 A354 A360 | A318 A331 A340 A363 | A344 A358 A361 A376 | A272 A274 A276 A286 A293 A298 A306 A309 | A268 A278 A302 A308 | A271 A283 A296 A303 | A265 A279 A281 A290 | A275 A300 A305 A313 | A277 A288 A292 A297 | A289 A294 A299 A312 | A237 A270 A287 A321 | A974 A981 A982 A983 A984 A1002 A1003 A1012 | A817 A823 A851 A856 | A65 A81 A82 A112 | A72 A78 A83 A100 | A24 A52 A58 A98 | A35 A49 A79 A97 | A14 A16 A59 A102 | A5 A7 A34 A51 | A9 A12 A15 A629 | A11 A57 A623 A627 | A8 A44 A46 A626 | A1 A10 A17 A18 A23 A26 A39 A42 | A1207 A1222 A1223 A1240 | A1201 A1221 A1225 A1242 | A221 A239 A1226 A1235 | A188 A219 A249 A258 | A222 A234 A243 A262 | A228 A229 A238 A253 | A232 A233 A248 A260 | A171 A182 A186 A211 | A1200 A1209 A1216 A1233 | A684 A702 A1292 A1293 | A1176 A1186 A1274 A1275 in component "Cover"
sketch "Sketch2" plane through (0, 0, 0) normal (0, 0, 1) x (1, 0, 0) in component "Cover"
  line L0 (6.4449, 24.826) -> (10.7371, 24.826)
  line L1 (10.7371, 24.826) -> (10.7371, 11.234)
  line L2 (10.7371, 11.234) -> (6.4449, 11.234)
  line L3 (6.4449, 11.234) -> (6.4449, 24.826)
  line L4 (22.8984, 35.6588) -> (51.0023, 35.6588)
  line L5 (51.0023, 35.6588) -> (51.0023, 28.8117)
  line L6 (51.0023, 28.8117) -> (22.8984, 28.8117)
  line L7 (22.8984, 28.8117) -> (22.8984, 35.6588)
  line L8 (70.0107, 33.9215) -> (80.3325, 33.9215)
  line L9 (80.3325, 33.9215) -> (80.3325, 28.8117)
  line L10 (80.3325, 28.8117) -> (70.0107, 28.8117)
  line L11 (70.0107, 28.8117) -> (70.0107, 33.9215)
  line L12 (109.8642, 24.5376) -> (115.4271, 24.5376)
  line L13 (115.4271, 24.5376) -> (115.4271, 11.234)
  line L14 (115.4271, 11.234) -> (109.8642, 11.234)
  line L15 (109.8642, 11.234) -> (109.8642, 24.5376)
  line L16 (77.5776, 14.2844) -> (86.1946, 14.2844)
  line L17 (86.1946, 14.2844) -> (86.1946, 2.5042)
  line L18 (86.1946, 2.5042) -> (77.5776, 2.5042)
  line L19 (77.5776, 2.5042) -> (77.5776, 14.2844)
  line L20 (8.2048, 8.3943) -> (46.1635, 8.3943)
  line L21 (46.1635, 8.3943) -> (46.1635, 2.5042)
  line L22 (46.1635, 2.5042) -> (8.2048, 2.5042)
  line L23 (8.2048, 2.5042) -> (8.2048, 8.3943)
  constraint horizontal L0
  constraint vertical L1
  constraint horizontal L2
  constraint vertical L3
  constraint horizontal L4
  constraint vertical L5
  constraint horizontal L6
  constraint vertical L7
  constraint horizontal L8
  constraint vertical L9
  constraint horizontal L10
  constraint vertical L11
  constraint horizontal L12
  constraint vertical L13
  constraint horizontal L14
  constraint vertical L15
  constraint horizontal L16
  constraint vertical L17
  constraint horizontal L18
  constraint vertical L19
  constraint horizontal L20
  constraint vertical L21
  constraint horizontal L22
  constraint vertical L23
extrude "Extrude2" cut sketch "Sketch2" along normal blind 2 from surface at -3.2 in component "Cover"
component "Cover" placed x (1, 0, 0) y (0, 1, 0) z (0, 0, 1) at (0, 0, 0)
